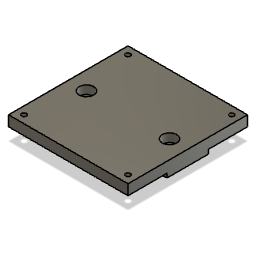
Vesa 100 x 100 Alu Profil 40x40 mount v2 (Autodesk Fusion 360 design; units mm, degrees)
Autodesk Fusion 360 part; units mm, degrees
note: some values were not read from the file. Set by a fixed rule: which sketch regions a step uses.
sketch "Sketch1" plane through (0, 0, 0) normal (0, 1, 0) x (1, 0, 0)
  line L0 (50, 50) -> (-50, 50)
  line L1 (-50, 50) -> (-50, -50)
  line L2 (-50, -50) -> (50, -50)
  line L3 (50, -50) -> (50, 50)
  line L4 (50, 50) -> (-50, -50) construction
  line L5 (-50, 50) -> (50, -50) construction
  circle A0 centre (-50, 50) radius 2.25
  circle A1 centre (50, 50) radius 2.25
  circle A2 centre (-50, -50) radius 2.25
  circle A3 centre (50, -50) radius 2.25
  line L6 (57.5, 57.5) -> (-57.5, 57.5)
  line L7 (-57.5, 57.5) -> (-57.5, -57.5)
  line L8 (-57.5, -57.5) -> (57.5, -57.5)
  line L9 (57.5, -57.5) -> (57.5, 57.5)
  line L10 (57.5, 57.5) -> (-57.5, -57.5) construction
  line L11 (-57.5, 57.5) -> (57.5, -57.5) construction
  circle A4 centre (-50, 50) radius 4
  circle A5 centre (50, 50) radius 4
  circle A6 centre (50, -50) radius 4
  circle A7 centre (-50, -50) radius 4
  dimension "d1" = 100
  dimension "d2" = 100
  dimension "d3" = 4.5
  dimension "d4" = 4.5
  dimension "d5" = 4.5
  dimension "d6" = 4.5
  dimension "d7" = 115
  dimension "d8" = 115
  dimension "d11" = 8
  dimension "d12" = 8
  dimension "d13" = 8
  dimension "d14" = 8
  constraint horizontal L0
  constraint perpendicular L0 L1
  constraint parallel L0 L2
  constraint parallel L1 L3
  constraint coincident L4 origin
  constraint coincident L5 origin
  constraint coincident L0.end L1.start
  constraint coincident L0.start L3.end
  constraint coincident L1.end L2.start
  constraint coincident L2.end L3.start
  constraint horizontal L6
  constraint perpendicular L6 L7
  constraint parallel L6 L8
  constraint parallel L7 L9
  constraint coincident L10 origin
  constraint coincident L11 origin
  constraint concentric A0 A4
  constraint concentric A1 A5
  constraint concentric A3 A6
  constraint concentric A2 A7
  measures "d1" distance of L1.end L2.end
  measures "d2" distance of L0.end L1.end
  measures "d3" diameter of A0
  measures "d4" diameter of A1
  measures "d5" diameter of A2
  measures "d6" diameter of A3
  measures "d7" distance of L7.end L8.end
  measures "d8" distance of L6.end L7.end
  measures "d11" diameter of A4
  measures "d12" diameter of A5
  measures "d13" diameter of A6
  measures "d14" diameter of A7
extrude "Extrude1" add sketch "Sketch1" along normal blind 10 contours L0 L1 A0 A4 | L0 L1 A0 A4 | L0 L1 L2 L3 A4 A5 A6 A7 | L0 L3 A1 A5 | L0 L3 A1 A5 | L1 L2 A2 A7 | L1 L2 A2 A7 | L2 L3 A3 A6 | L2 L3 A3 A6 | L6 L7 L8 L9
extrude "Extrude2" cut sketch "Sketch1" along normal blind 6 contours L0 L1 A0 A4 | L0 L1 A0 A4 | L0 L3 A1 A5 | L0 L3 A1 A5 | L1 L2 A2 A7 | L1 L2 A2 A7 | L2 L3 A3 A6 | L2 L3 A3 A6
sketch "Sketch2" plane through (0, 0, 0) normal (0, 1, 0) x (1, 0, 0)
  line L0 (57.5, 20) -> (-57.5, 20)
  line L1 (-57.5, 20) -> (-57.5, -20)
  line L2 (-57.5, -20) -> (57.5, -20)
  line L3 (57.5, -20) -> (57.5, 20)
  line L4 (57.5, 20) -> (-57.5, -20) construction
  line L5 (-57.5, 20) -> (57.5, -20) construction
  dimension "d17" = 115
  dimension "d18" = 40
  constraint horizontal L0
  constraint perpendicular L0 L1
  constraint parallel L0 L2
  constraint parallel L1 L3
  constraint coincident L4 origin
  constraint coincident L5 origin
  measures "d17" distance of L1.end L2.end
  measures "d18" distance of L0.end L1.end
extrude "Extrude3" add sketch "Sketch2" against normal blind 20
sketch "Sketch3" plane through (0, 10, 0) normal (0, 1, 0) x (-1, 0, 0)
  circle A0 centre (50, -50) radius 2.25
  circle A1 centre (-50, -50) radius 2.25
  circle A2 centre (-50, 50) radius 2.25
  circle A3 centre (50, 50) radius 2.25
  line L0 (-57.5, 57.5) -> (-57.5, -57.5)
  line L1 (-57.5, -57.5) -> (57.5, -57.5)
  line L2 (57.5, -57.5) -> (57.5, 57.5)
  line L3 (57.5, 57.5) -> (-57.5, 57.5)
  circle A4 centre (-40, 0) radius 7
  circle A5 centre (40, 0) radius 7
  circle A6 centre (40, 0) radius 4.25
  circle A7 centre (-40, 0) radius 4.25
  dimension "d21" = 14
  dimension "d22" = 14
  dimension "d23" = 8.5
  dimension "d24" = 8.5
  constraint concentric A5 A6
  constraint concentric A4 A7
  measures "d21" diameter of A4
  measures "d22" diameter of A5
  measures "d23" diameter of A6
  measures "d24" diameter of A7
extrude "Extrude4" cut sketch "Sketch3" against normal blind 8 contours A4 | A5
extrude "Extrude5" cut 2 faces at (-40.8833, 10, 1.9427) (39.1167, 10, 1.9427) along direction (0, -1, 0) blind 37
extrude "Extrude6" cut 1 faces at (-12.625, -20, 14.5602) along direction (0, 1, 0) blind 15
extrude "Extrude7" cut 1 faces at (-12.625, -5, 14.5602) along direction (0, 1, 0) blind 1
sketch "Sketch4" plane through (0, -4, 0) normal (0, -1, 0) x (1, 0, 0)
  circle A0 centre (-40, 0) radius 4.25
  circle A1 centre (40, 0) radius 4.25
  line L0 (57.5, -20) -> (57.5, 20)
  line L1 (57.5, 20) -> (-57.5, 20)
  line L2 (-57.5, 20) -> (-57.5, -20)
  line L3 (-57.5, -20) -> (57.5, -20)
  line L4 (-22, 5) -> (-32, 5)
  line L5 (-32, 5) -> (-32, -5)
  line L6 (-32, -5) -> (-22, -5)
  line L7 (-22, -5) -> (-22, 5)
  line L8 (-22, 5) -> (-32, -5) construction
  line L9 (-32, 5) -> (-22, -5) construction
  line L10 (0, 1.75) -> (0, 22.5)
  line L11 (22, 5) -> (32, 5)
  line L12 (32, 5) -> (32, -5)
  line L13 (32, -5) -> (22, -5)
  line L14 (22, -5) -> (22, 5)
  point P0 (-27, 0)
  dimension "d33" = 10
  dimension "d34" = 10
  constraint horizontal L4
  constraint perpendicular L4 L5
  constraint parallel L4 L6
  constraint parallel L5 L7
  constraint coincident L8 P0
  constraint coincident L9 P0
  constraint symmetric L4.start L10 L11.start
  constraint symmetric L4.end L10 L11.end
  constraint symmetric L5.end L10 L12.end
  constraint symmetric L6.end L10 L13.end
  measures "d33" distance of L5.end L6.end
  measures "d34" distance of L4.end L5.end
extrude "Extrude8" add sketch "Sketch4" along normal blind 8 contours L4 L5 L6 L7 | L11 L12 L13 L14
